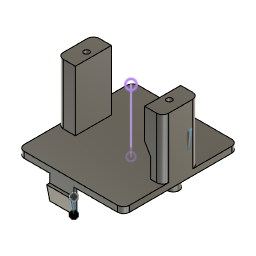
Gruppo-sonar v6 (Autodesk Fusion 360 archive; units mm, degrees)
design "Supporto-SG90"
Autodesk Fusion 360 part; units mm, degrees
sketch "Schizzo1" plane through (0, 0, 0) normal (0, 0, 1) x (1, 0, 0)
  line L0 (-15, 20) -> (27, 20)
  line L1 (27, 20) -> (27, -20)
  line L2 (27, -20) -> (-15, -20)
  line L3 (-15, -20) -> (-15, 20)
  circle A0 centre (0, 0) radius 9.75
  circle A1 centre (22, 0) radius 2
  line L4 (0, 0) -> (22, 0) construction
  dimension "d1" = 19.5
  dimension "d4" = 4
  dimension "d5" = 22
  dimension "d6" = 15
  dimension "d8" = 5
  dimension "d9" = 20
  dimension "d10" = 20
  constraint horizontal L0
  constraint vertical L1
  constraint horizontal L2
  constraint vertical L3
  constraint coincident A0.centre L4.start
  constraint coincident A1.centre L4.end
  constraint horizontal L4
  measures "d1" diameter of A0
  measures "d4" diameter of A1
  measures "d5" distance of A0.centre A1.centre
  measures "d6" distance of L3 A0.centre
  measures "d8" distance of L1 A1.centre
  measures "d9" distance of A0.centre L0
  measures "d10" distance of A0.centre L2
extrude "Estrusione1" add sketch "Schizzo1" along normal blind 2.5 contours A0 | A1 makes body 1 at (-1.7521, -4.8561, 0) makes body 2 at (23.9975, -0.0997, 1.6667)
sketch "Schizzo2" plane through (0, 0, 2.5) normal (0, 0, 1) x (-1, 0, 0)
  circle A0 centre (0, 0) radius 9.75
  line L0 (0, -19) -> (-8, -19)
  line L1 (-8, -19) -> (-8, -18)
  line L2 (-8, -18) -> (0, -18)
  line L3 (0, -18) -> (0, -19)
  line L4 (0, 18) -> (-8, 18)
  line L5 (-8, 18) -> (-8, 19)
  line L6 (-8, 19) -> (0, 19)
  line L7 (0, 19) -> (0, 18)
  line L8 (0, -18) -> (0, 0) construction
  line L9 (0, 0) -> (0, 18) construction
  dimension "d14" = 38
  dimension "d15" = 1
  dimension "d16" = 8
  constraint horizontal L0
  constraint vertical L1
  constraint horizontal L2
  constraint vertical L3
  constraint horizontal L4
  constraint vertical L5
  constraint horizontal L6
  constraint vertical L7
  constraint coincident A0.centre L8.end
  constraint perpendicular L2 L8
  constraint perpendicular L4 L9
  constraint equal L8 L9
  constraint equal L1 L5
  constraint equal L2 L4
  measures "d14" distance of L0 L6
  measures "d15" distance of L0.end L1.end
  measures "d16" distance of L0.start L0.end
extrude "Estrusione2" add sketch "Schizzo2" against normal blind 8 separate body contours L0 L1 L2 L3 | L4 L5 L6 L7 makes body 3 at (2.6667, 19, -0.1667) makes body 4 at (2.6667, -19, -2.8333)
sketch "Schizzo3" plane through (8, 0, 0) normal (1, 0, 0) x (0, 1, 0)
  line L0 (-18, 2.5) -> (-19, 2.5)
  line L1 (-19, 2.5) -> (-19, -5.5)
  line L2 (-19, -5.5) -> (-18, -5.5)
  line L3 (-18, -5.5) -> (-18, 2.5)
  line L4 (-19, -5.5) -> (-20, -0.332)
  line L5 (-20, -0.332) -> (-19, -0.332)
  line L6 (0, 1.75) -> (0, 22.5)
  line L7 (20, -0.332) -> (19, -0.332)
  line L8 (19, -5.5) -> (20, -0.332)
  line L9 (19, -0.332) -> (19, -5.5)
  dimension "d21" = 1
  constraint coincident L1.end L2.start
  constraint perpendicular L1 L5
  constraint coincident L1 L5.end
  constraint symmetric L1.end L6 L8.start
  constraint symmetric L4.end L6 L7.start
  constraint symmetric L5.end L6 L7.end
  measures "d21" distance of L4.end L5.end
extrude "Estrusione4" add sketch "Schizzo3" against normal up to surface (8 mm away) contours L1 L4 L5 | L7 L8 L9 bodies 3 4
sketch "Schizzo4" plane through (0, 0, 2.5) normal (0, 0, 1) x (-1, 0, 0)
  circle A0 centre (0, 0) radius 9.75
  line L0 (10.5, -19) -> (-24.5, -19)
  line L1 (-24.5, -19) -> (-24.5, 19)
  line L2 (-24.5, 19) -> (10.5, 19)
  line L3 (10.5, 19) -> (10.5, -19)
  line L4 (0, -19) -> (-8, -19)
  line L5 (-8, 19) -> (0, 19)
  dimension "d25" = 35
  dimension "d26" = 10.5
  constraint horizontal L0
  constraint vertical L1
  constraint horizontal L2
  constraint vertical L3
  constraint collinear L0 L4
  constraint collinear L2 L5
  measures "d25" distance of L0.start L0.end
  measures "d26" distance of A0.centre L3
extrude "Estrusione5" add sketch "Schizzo4" along normal blind 2 contours A0 | L0 L1 L2 L3 L4 L5 bodies 1 2 3 4
sketch "Schizzo5" plane through (0, 0, 4.5) normal (0, 0, 1) x (-1, 0, 0)
  line L0 (10.5, 19) -> (-24.5, 19)
  line L1 (-24.5, 19) -> (-24.5, -19)
  line L2 (-24.5, -19) -> (10.5, -19)
  line L3 (10.5, -19) -> (10.5, 19)
  line L4 (10.5, -6) -> (4.5, -6)
  line L5 (4.5, -6) -> (4.5, 6)
  line L6 (4.5, 6) -> (10.5, 6)
  line L7 (10.5, 6) -> (10.5, -6)
  line L8 (-24.5, -6) -> (-18.5, -6)
  line L9 (-18.5, -6) -> (-18.5, 6)
  line L10 (-18.5, 6) -> (-24.5, 6)
  line L11 (-24.5, 6) -> (-24.5, -6)
  line L12 (4.5, -6) -> (0, 0) construction
  line L13 (0, 0) -> (4.5, 6) construction
  dimension "d29" = 23
  dimension "d30" = 12
  constraint horizontal L4
  constraint vertical L5
  constraint horizontal L6
  constraint vertical L7
  constraint horizontal L8
  constraint vertical L9
  constraint horizontal L10
  constraint vertical L11
  constraint collinear L1 L11
  constraint collinear L3 L7
  constraint collinear L4 L8
  constraint collinear L6 L10
  constraint equal L4 L8
  constraint coincident L12.end L13.start
  constraint equal L12 L13
  measures "d29" distance of L5 L9
  measures "d30" distance of L4.start L6.end
extrude "Estrusione6" add sketch "Schizzo5" along normal blind 20 contours L3 L4 L5 L6 L7 | L1 L8 L9 L10 L11 bodies 1
sketch "Schizzo6" plane through (0, -6, 0) normal (0, -1, 0) x (1, 0, 0)
  line L0 (18.5, 4.5) -> (24.5, 4.5)
  line L1 (24.5, 4.5) -> (24.5, 24.5)
  line L2 (24.5, 24.5) -> (18.5, 24.5)
  line L3 (18.5, 24.5) -> (18.5, 4.5)
  line L4 (18.5, 14.5) -> (20.5, 11.0359)
  line L5 (20.5, 11.0359) -> (20.5, 4.5)
  line L6 (20.5, 4.5) -> (18.5, 4.5)
  line L7 (18.5, 4.5) -> (18.5, 14.5)
  line L8 (-10.5, 4.5) -> (24.5, 4.5)
  dimension "d33" = 10
  dimension "d34" = 2
  dimension "d35" = 30
  constraint parallel L3 L5
  constraint perpendicular L3 L6
  constraint collinear L6 L8
  constraint vertical L7
  constraint collinear L3 L7
  constraint coincident L3 L4.start
  measures "d33" distance of L4.start L0.start
  measures "d34" distance of L5 L7
  measures "d35" angle of L4 L7
extrude "Estrusione7" cut sketch "Schizzo6" against normal through all contours L0 L3 L4 L5 L6 L7 L8 bodies 1
sketch "Schizzo7" plane through (0, 0, 24.5) normal (0, 0, 1) x (-1, 0, 0)
  line L0 (10.5, 6) -> (4.5, 6)
  line L1 (4.5, 6) -> (4.5, -6)
  line L2 (4.5, -6) -> (10.5, -6)
  line L3 (10.5, -6) -> (10.5, 6)
  line L4 (6.75, 0) -> (-20.75, 0)
  line L5 (6.75, 0) -> (10.5, 0)
  line L6 (-20.75, 0) -> (-24.5, 0)
  line L7 (-24.5, 6) -> (-24.5, -6)
  point P0 (6.75, 0)
  point P1 (-20.75, 0)
  dimension "d37" = 27.5
  constraint perpendicular L3 L4
  constraint midpoint L3 L5.end
  constraint midpoint L6.end L7
  constraint equal L5 L6
  constraint coincident P0 L4.start
  constraint coincident P1 L4.end
  constraint collinear L4 L6
  measures "d37" distance of P0 P1
hole "Foratura1" at (-6.75, 0, 24.5) at (20.75, 0, 24.5) direction (0, 0, -1) diameter 1.8 depth 10 tip angle 118 bodies 1
fillet "Raccordo1" radius 2 8 edges at (-10.5, -6, 14.5) (-10.5, 6, 14.5) (24.5, -6, 14.5) (24.5, 6, 14.5) (24.5, -19, 3.5) (-10.5, -19, 3.5) (-10.5, 19, 3.5) (24.5, 19, 3.5) on bodies 1

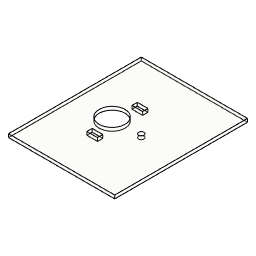
design "Ripiano-Smart-car"
Autodesk Fusion 360 part; units mm, degrees
sketch "Schizzo1" plane through (0, 0, 0) normal (0, 0, 1) x (1, 0, 0)
  line L0 (-80, 50) -> (0, 50)
  line L1 (0, 50) -> (0, -50)
  line L2 (0, -50) -> (-80, -50)
  line L3 (-80, -50) -> (-80, 50)
  dimension "d1" = 100
  dimension "d2" = 80
  constraint horizontal L0
  constraint vertical L1
  constraint horizontal L2
  constraint vertical L3
  constraint midpoint origin L1
  measures "d1" distance of L0.start L2.end
  measures "d2" distance of L0.start L0.end
extrude "Estrusione1" add sketch "Schizzo1" along normal blind 2.5
sketch "Schizzo2" plane through (0, 0, 2.5) normal (0, 0, 1) x (-1, 0, 0)
  line L0 (80, 50) -> (0, 50)
  line L1 (0, 50) -> (0, -50)
  line L2 (0, -50) -> (80, -50)
  line L3 (80, -50) -> (80, 50)
  line L4 (0, 0) -> (30, 0)
  line L5 (30, 0) -> (52, 0)
  point P0 (52, 0)
  point P1 (30, 0)
  dimension "d8" = 30
  dimension "d9" = 22
  constraint horizontal P0 P1
  constraint coincident L4.start origin
  constraint perpendicular L3 L4
  constraint coincident P1 L4.end
  constraint coincident P0 L5.end
  measures "d8" distance of L4.start P1
  measures "d9" distance of P1 P0
hole "Foratura1" at (-52, 0, 2.5) direction (0, 0, -1) diameter 19.5 end through all
hole "Foratura2" at (-30, 0, 2.5) direction (0, 0, -1) diameter 4 end through all
sketch "Schizzo3" plane through (0, 0, 2.5) normal (0, 0, 1) x (-1, 0, 0)
  circle A0 centre (30, 0) radius 2
  circle A1 centre (52, 0) radius 9.75
  line L0 (80, 50) -> (0, 50)
  line L1 (0, 50) -> (0, -50)
  line L2 (0, -50) -> (80, -50)
  line L3 (80, -50) -> (80, 50)
  line L4 (52, -19) -> (44, -19)
  line L5 (44, -19) -> (44, -15)
  line L6 (44, -15) -> (52, -15)
  line L7 (52, -15) -> (52, -19)
  line L8 (52, 15) -> (44, 15)
  line L9 (44, 15) -> (44, 19)
  line L10 (44, 19) -> (52, 19)
  line L11 (52, 19) -> (52, 15)
  line L12 (44, -15) -> (0, 0) construction
  line L13 (44, 15) -> (0, 0) construction
  line L14 (44, -15) -> (44, 15) construction
  dimension "d13" = 4
  dimension "d14" = 8
  dimension "d15" = 30
  dimension "d16" = 52
  constraint horizontal L4
  constraint vertical L5
  constraint horizontal L6
  constraint vertical L7
  constraint horizontal L8
  constraint vertical L9
  constraint horizontal L10
  constraint vertical L11
  constraint equal L6 L8
  constraint equal L5 L9
  constraint coincident L12.end L13.end
  constraint vertical L14
  constraint equal L12 L13
  measures "d13" distance of L4.start L6.end
  measures "d14" distance of L4.start L4.end
  measures "d15" distance of L6 L8
  measures "d16" distance of L1 L7
extrude "Estrusione2" cut sketch "Schizzo3" against normal through all contours L4 L5 L6 L7 | L8 L9 L10 L11
